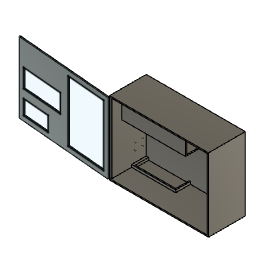
Dispenser (Autodesk Fusion 360 design; units mm, degrees)
Autodesk Fusion 360 part; units mm, degrees
note: some values were not read from the file. Chosen so that the rebuilt part matches the saved one: which bodies a step acts on. Set by a fixed rule: which sketch regions a step uses.
sketch "Sketch1" plane through (0, 0, 0) normal (0, 0, 1) x (1, 0, 0) in component "Box"
  line L0 (0, 0) -> (-404, 0)
  line L1 (-404, 0) -> (-404, 150)
  line L2 (-404, 150) -> (0, 150)
  line L3 (0, 150) -> (0, 0)
  dimension "d1" = 404
  dimension "d2" = 150
  constraint horizontal L0
  constraint vertical L1
  constraint horizontal L2
  constraint vertical L3
  constraint coincident L0.start L3.end
  measures "d1" distance of L0.start L0.end
  measures "d2" distance of L0.start L2.end
extrude "Extrude1" add sketch "Sketch1" along normal blind 298 makes body 1 in component "Box"
shell "Shell1" thickness 5 removed faces 0 bodies 1 in component "Box"
ref_plane "WorkPlane1" through (-202, 5, 149) normal (0, -1, 0) x (1, 0, 0) in component "Box"
split "Split1" by plane through (-202, 5, 149) normal (0, -1, 0) bodies 1 makes body 2 at (-134.6667, 0, 99.3333) in component "Box"
ref_plane "WorkPlane2" through (-202, 75, 293) normal (0, 0, 1) x (1, 0, 0) in component "Box"
ref_plane "WorkPlane3" through (-202, 75, 5) normal (0, 0, -1) x (-1, 0, 0) in component "Box"
ref_plane "WorkPlane4" through (-5, 75, 149) normal (1, 0, 0) x (0, 1, 0) in component "Box"
split "Split2" by plane through (-202, 75, 293) normal (0, 0, 1) and through (-202, 75, 5) normal (0, 0, -1) bodies 2 makes body 3 at (-136.3333, 5, 296.3333) makes body 4 at (-134.6667, 0, 1.6667) in component "Box"
split "Split3" by plane through (-5, 75, 149) normal (1, 0, 0) bodies 2 makes body 5 at (-1.6667, 5, 197) in component "Box"
combine "Combine1" operation add target body 1 tool bodies 3 5 4 in component "Box"
move_body "Move1" bodies 2 to x (-0.996195, 0.087156, 0) y (-0.087156, -0.996195, 0) z (0, 0, 1) at (-806.4627, 35.2109, 0) in component "Box"
sketch "Sketch3" plane through (-3.5046, -40.0579, 0) normal (-0.087156, -0.996195, 0) x (0.996195, -0.087156, 0) in component "Box"
  line L0 (-801.4627, 293) -> (-801.4627, 5)
  line L1 (-801.4627, 5) -> (-402.4627, 5)
  line L2 (-402.4627, 5) -> (-402.4627, 293)
  line L3 (-402.4627, 293) -> (-801.4627, 293)
  line L4 (-581.4627, 273) -> (-422.4627, 273)
  line L5 (-422.4627, 273) -> (-422.4627, 25)
  line L6 (-422.4627, 25) -> (-581.4627, 25)
  line L7 (-581.4627, 25) -> (-581.4627, 273)
  line L8 (-781.4627, 120) -> (-616.4627, 120)
  line L9 (-616.4627, 120) -> (-616.4627, 195)
  line L10 (-616.4627, 195) -> (-781.4627, 195)
  line L11 (-781.4627, 195) -> (-781.4627, 120)
  line L12 (-781.4627, 85) -> (-671.4627, 85)
  line L13 (-671.4627, 85) -> (-671.4627, 25)
  line L14 (-671.4627, 25) -> (-781.4627, 25)
  line L15 (-781.4627, 25) -> (-781.4627, 85)
  dimension "d23" = 159
  dimension "d24" = 248
  dimension "d25" = 165
  dimension "d26" = 75
  dimension "d28" = 20
  dimension "d31" = 20
  dimension "d32" = 20
  dimension "d33" = 110
  dimension "d34" = 60
  dimension "d35" = 20
  dimension "d37" = 20
  dimension "d38" = 35
  constraint horizontal L4
  constraint vertical L5
  constraint horizontal L6
  constraint vertical L7
  constraint horizontal L8
  constraint vertical L9
  constraint horizontal L10
  constraint vertical L11
  constraint horizontal L12
  constraint vertical L13
  constraint horizontal L14
  constraint vertical L15
  measures "d23" distance of L4.start L4.end
  measures "d24" distance of L4.start L6.end
  measures "d25" distance of L8.start L8.end
  measures "d26" distance of L8.start L10.end
  measures "d28" distance of L3 L4
  measures "d31" distance of L0 L11
  measures "d32" distance of L2 L5
  measures "d33" distance of L12.start L12.end
  measures "d34" distance of L12.start L14.end
  measures "d35" distance of L0 L15
  measures "d37" distance of L1 L14
  measures "d38" distance of L8 L12
extrude "Extrude2" cut sketch "Sketch3" against normal up to surface (5 mm away) contours L4 L5 L6 L7 bodies 2 in component "Box"
extrude "Extrude3" cut sketch "Sketch3" against normal up to surface (5 mm away) contours L8 L9 L10 L11 | L12 L13 L14 L15 bodies 2 in component "Box"
sketch "Sketch4" plane through (-399, 0, 0) normal (1, 0, 0) x (0, 1, 0) in component "Box"
  line L0 (5, 5) -> (145, 5)
  line L1 (145, 5) -> (145, 293)
  line L2 (145, 293) -> (5, 293)
  line L3 (5, 293) -> (5, 5)
  line L4 (145, 198) -> (45, 198)
  line L5 (45, 198) -> (45, 193)
  line L6 (45, 193) -> (145, 193)
  line L7 (145, 193) -> (145, 198)
  line L8 (150, 298) -> (0, 298)
  dimension "d44" = 5
  dimension "d45" = 100
  dimension "d46" = 100
  constraint horizontal L4
  constraint vertical L5
  constraint horizontal L6
  constraint vertical L7
  measures "d44" distance of L4.start L6.end
  measures "d45" distance of L4 L8
  measures "d46" distance of L1 L4.end
extrude "Extrude4" add sketch "Sketch4" along normal blind 280 separate body contours L1 L4 L5 L6 L7 makes body 6 in component "Box"
combine "Combine2" operation add target body 1 tool bodies 6 in component "Box"
sketch "Sketch5" plane through (0, 0, 5) normal (0, 0, 1) x (-1, 0, 0) in component "Box"
  line L0 (5, -145) -> (399, -145)
  line L1 (399, -145) -> (399, -5)
  line L2 (399, -5) -> (404, -5)
  line L3 (404, -5) -> (404, 0)
  line L4 (404, 0) -> (5, 0)
  line L5 (5, 0) -> (5, -145)
  line L6 (399, -145) -> (389, -145)
  line L7 (399, -85) -> (389, -85)
  line L8 (389, -85) -> (219, -85)
  line L9 (219, -85) -> (219, -145)
  line L10 (224, -145) -> (224, -90)
  line L11 (224, -90) -> (389, -90)
  line L12 (389, -90) -> (389, -145)
  dimension "d52" = 10
  dimension "d53" = 60
  dimension "d54" = 170
  dimension "d55" = 5
  constraint coincident L0.end L1.start
  constraint perpendicular L1 L6
  constraint coincident L1 L7.start
  constraint perpendicular L1 L7
  constraint coincident L0 L9.end
  constraint perpendicular L0 L9
  constraint coincident L0 L10.start
  constraint perpendicular L0 L10
  constraint perpendicular L6 L12
  measures "d52" distance of L0.end L6.end
  measures "d53" distance of L6.end L7.end
  measures "d54" distance of L7.end L8.end
  measures "d55" distance of L9 L10
extrude "Extrude5" add sketch "Sketch5" along normal blind 10 contours L0 L1 L6 L7 L8 L9 L10 L11 L12 bodies 1 in component "Box"
sketch "Sketch6" plane through (-399, 0, 0) normal (1, 0, 0) x (0, 1, 0) in component "Box"
  line L0 (85, 15) -> (145, 15)
  line L1 (145, 15) -> (145, 193)
  line L2 (145, 193) -> (45, 193)
  line L3 (45, 193) -> (45, 198)
  line L4 (45, 198) -> (145, 198)
  line L5 (145, 198) -> (145, 293)
  line L6 (145, 293) -> (5, 293)
  line L7 (5, 293) -> (5, 5)
  line L8 (5, 5) -> (85, 5)
  line L9 (85, 5) -> (85, 15)
  line L10 (105, 30) -> (95, 30)
  line L11 (95, 30) -> (95, 20)
  line L12 (95, 20) -> (105, 20)
  line L13 (105, 20) -> (105, 30)
  line L14 (95, 90) -> (130, 90)
  line L15 (130, 90) -> (130, 58)
  line L16 (130, 58) -> (95, 58)
  line L17 (95, 58) -> (95, 90)
  line L18 (130, 90) -> (128, 90)
  line L19 (128, 90) -> (128, 88)
  line L20 (128, 88) -> (130, 88)
  line L21 (130, 88) -> (130, 90)
  circle A0 centre (128, 88) radius 1
  line L22 (95, 90) -> (97, 90)
  line L23 (97, 90) -> (97, 88)
  line L24 (97, 88) -> (95, 88)
  line L25 (95, 88) -> (95, 90)
  line L26 (95, 58) -> (97, 58)
  line L27 (97, 58) -> (97, 60)
  line L28 (97, 60) -> (95, 60)
  line L29 (95, 60) -> (95, 58)
  line L30 (130, 58) -> (128, 58)
  line L31 (128, 58) -> (128, 60)
  line L32 (128, 60) -> (130, 60)
  line L33 (130, 60) -> (130, 58)
  circle A1 centre (97, 88) radius 1
  circle A2 centre (97, 60) radius 1
  circle A3 centre (128, 60) radius 1
  dimension "d58" = 10
  dimension "d59" = 10
  dimension "d61" = 25
  dimension "d62" = 40
  dimension "d63" = 35
  dimension "d64" = 32
  dimension "d65" = 50
  dimension "d66" = 2
  dimension "d67" = 2
  dimension "d68" = 2
  dimension "d70" = 2
  dimension "d71" = 2
  dimension "d72" = 2
  dimension "d73" = 2
  dimension "d74" = 2
  dimension "d75" = 2
  dimension "d76" = 2
  dimension "d77" = 2
  dimension "d78" = 2
  constraint horizontal L10
  constraint vertical L11
  constraint horizontal L12
  constraint vertical L13
  constraint horizontal L14
  constraint vertical L15
  constraint horizontal L16
  constraint vertical L17
  constraint horizontal L18
  constraint vertical L19
  constraint horizontal L20
  constraint vertical L21
  constraint coincident L19.end L20.start
  constraint horizontal L22
  constraint vertical L23
  constraint horizontal L24
  constraint vertical L25
  constraint horizontal L26
  constraint vertical L27
  constraint horizontal L28
  constraint vertical L29
  constraint horizontal L30
  constraint vertical L31
  constraint horizontal L32
  constraint vertical L33
  constraint coincident L23.end L24.start
  constraint coincident L27.end L28.start
  constraint coincident L31.end L32.start
  measures "d58" distance of L10.start L10.end
  measures "d59" distance of L10.start L12.end
  measures "d61" distance of L8 L10
  measures "d62" distance of L1 L13
  measures "d63" distance of L14.start L14.end
  measures "d64" distance of L14.start L16.end
  measures "d65" distance of L1 L17
  measures "d66" distance of L14.end L18.end
  measures "d67" distance of L14.end L20.end
  measures "d68" diameter of A0
  measures "d70" distance of L14.start L22.end
  measures "d71" distance of L14.start L24.end
  measures "d72" distance of L16.end L26.end
  measures "d73" distance of L16.end L28.end
  measures "d74" distance of L15.end L30.end
  measures "d75" distance of L15.end L32.end
  measures "d76" diameter of A1
  measures "d77" diameter of A2
  measures "d78" diameter of A3
extrude "Extrude6" add sketch "Sketch6" along normal blind 5 contours L23 L24 A1 | L23 L24 A1 | L19 L20 A0 | L19 L20 A0 | L27 L28 A2 | L27 L28 A2 | L31 L32 A3 | L31 L32 A3 bodies 1 in component "Box"
sketch "Sketch7" plane through (0, 0, 193) normal (0, 0, -1) x (1, 0, 0) in component "Box"
  line L0 (-399, -45) -> (-399, -145)
  line L1 (-399, -145) -> (-119, -145)
  line L2 (-119, -145) -> (-119, -45)
  line L3 (-119, -45) -> (-399, -45)
  line L4 (-389, -90) -> (-382, -90)
  line L5 (-382, -90) -> (-382, -100)
  line L6 (-382, -100) -> (-389, -100)
  line L7 (-389, -100) -> (-389, -90)
  dimension "d81" = 7
  dimension "d82" = 10
  dimension "d83" = 45
  dimension "d84" = 10
  constraint horizontal L4
  constraint vertical L5
  constraint horizontal L6
  constraint vertical L7
  measures "d81" distance of L4.start L4.end
  measures "d82" distance of L4.start L6.end
  measures "d83" distance of L3 L4
  measures "d84" distance of L0 L7
sketch "Sketch8" plane through (0, 0, 198) normal (0, 0, 1) x (-1, 0, 0) in component "Box"
  line L0 (399, -145) -> (399, -45)
  line L1 (399, -45) -> (119, -45)
  line L2 (119, -45) -> (119, -145)
  line L3 (119, -145) -> (399, -145)
  line L4 (399, -145) -> (381, -145)
  line L5 (381, -145) -> (381, -45)
  line L6 (381, -45) -> (399, -45)
  line L7 (399, -45) -> (399, -145)
  dimension "d86" = 18
  dimension "d87" = 100
  constraint horizontal L4
  constraint vertical L5
  constraint horizontal L6
  constraint vertical L7
  constraint coincident L0.start L3.end
  measures "d86" distance of L0.start L4.end
  measures "d87" distance of L0.start L0.end
extrude "Extrude7" cut sketch "Sketch7" against normal up to surface (5 mm away) contours L4 L5 L6 L7 bodies 1 in component "Box"
extrude "Extrude8" add sketch "Sketch8" along normal blind 35 contours L0 L1 L3 L4 L5 L6 L7 bodies 1 in component "Box"
sketch "Sketch9" plane through (-381, 0, 0) normal (1, 0, 0) x (0, 1, 0) in component "Box"
  line L0 (45, 198) -> (145, 198)
  line L1 (145, 198) -> (145, 233)
  line L2 (145, 233) -> (45, 233)
  line L3 (45, 233) -> (45, 198)
  circle A0 centre (95, 215) radius 14
  line L4 (87.7, 198) -> (102.3, 198)
  line L5 (102.3, 198) -> (102.3, 203)
  line L6 (102.3, 203) -> (87.7, 203)
  line L7 (87.7, 203) -> (87.7, 198)
  dimension "d92" = 28
  dimension "d93" = 50
  dimension "d94" = 17
  dimension "d95" = 14.6
  dimension "d96" = 5
  dimension "d97" = 42.7
  constraint horizontal L4
  constraint vertical L5
  constraint horizontal L6
  constraint vertical L7
  constraint coincident L0 L4.start
  measures "d92" diameter of A0
  measures "d93" distance of L1 A0.centre
  measures "d94" distance of L0 A0.centre
  measures "d95" distance of L4.start L4.end
  measures "d96" distance of L4.start L6.end
  measures "d97" distance of L1 L5
extrude "Extrude9" cut sketch "Sketch9" against normal up to surface (18 mm away) contours L0 A0 L4 L5 L6 L7 | A0 L6 | A0 L6 bodies 1 in component "Box"
sketch "Sketch10" plane through (0, 0, 198) normal (0, 0, 1) x (-1, 0, 0) in component "Box"
  line L0 (389, -90) -> (389, -100)
  line L1 (389, -100) -> (382, -100)
  line L2 (382, -100) -> (382, -90)
  line L3 (382, -90) -> (389, -90)
  line L4 (381, -145) -> (381, -102.3)
  line L5 (381, -102.3) -> (399, -102.3)
  line L6 (399, -102.3) -> (399, -87.7)
  line L7 (399, -87.7) -> (381, -87.7)
  line L8 (381, -87.7) -> (381, -45)
  line L9 (381, -45) -> (119, -45)
  line L10 (119, -45) -> (119, -145)
  line L11 (119, -145) -> (381, -145)
  line L12 (381, -45) -> (119, -45)
  line L13 (119, -45) -> (119, -50)
  line L14 (119, -50) -> (381, -50)
  line L15 (381, -50) -> (381, -45)
  dimension "d100" = 5
  constraint horizontal L12
  constraint vertical L13
  constraint horizontal L14
  constraint vertical L15
  constraint coincident L8.end L9.start
  measures "d100" distance of L8.end L14.end
extrude "Extrude10" add sketch "Sketch10" along normal up to surface (35 mm away) contours L8 L9 L10 L12 L13 L14 L15 bodies 1 in component "Box"
move_face "OffsetFaces1" offset -20 1 faces at (-119, 80, 194.6667) on bodies 1 in component "Box"
move_face "OffsetFaces2" offset 15 1 faces at (-393, 80, 233) on bodies 1 in component "Box"
extrude "Extrude11" add 1 faces at (-399, 92.9024, 212.4305) along direction (1, 0, 0) blind 18 on bodies 1 bodies 1 in component "Box"
sketch "Sketch11" plane through (-381, 0, 0) normal (1, 0, 0) x (0, 1, 0) in component "Box"
  line L0 (50, 198) -> (145, 198)
  line L1 (145, 198) -> (145, 248)
  line L2 (145, 248) -> (50, 248)
  line L3 (50, 248) -> (50, 198)
  circle A0 centre (95, 230) radius 14
  line L4 (87.7, 218) -> (102.3, 218)
  line L5 (102.3, 218) -> (102.3, 213)
  line L6 (102.3, 213) -> (87.7, 213)
  line L7 (87.7, 213) -> (87.7, 218)
  dimension "d107" = 28
  dimension "d108" = 50
  dimension "d109" = 32
  dimension "d110" = 14.6
  dimension "d111" = 5
  dimension "d112" = 42.7
  dimension "d113" = 15
  constraint horizontal L4
  constraint vertical L5
  constraint horizontal L6
  constraint vertical L7
  measures "d107" diameter of A0
  measures "d108" distance of L1 A0.centre
  measures "d109" distance of L0 A0.centre
  measures "d110" distance of L4.start L4.end
  measures "d111" distance of L4.start L6.end
  measures "d112" distance of L1 L5
  measures "d113" distance of L0 L6
extrude "Extrude12" cut sketch "Sketch11" against normal up to surface (18 mm away) contours A0 L4 | A0 L4 | A0 L4 L5 L6 L7 bodies 1 in component "Box"
extrude "Extrude13" cut 1 faces at (-384.3333, 93.3333, 198) along direction (0, 0, 1) up to surface (15 mm away) on bodies 1 bodies 1 in component "Box"
component "Box" placed x (1, 0, 0) y (0, 1, 0) z (0, 0, 1) at (4.5931, -0.4018, -1.729)
equation "d1 = BoxLength"
equation "d2 = BoxWidth"
equation "BoxHeight = 298 mm"
equation "WallThickness = 5 mm"
equation "BoxWidth = 150 mm"
equation "BoxLength = 404 mm"
equation "d7 = BoxHeight"
equation "d9 = WallThickness"
equation "d10 = -WallThickness"
equation "d11 = -WallThickness"
equation "d12 = -WallThickness"
equation "d13 = -WallThickness"
equation "HingeRadius = HingeThickness * 2"
equation "Gap = HingeThickness * 0.5 / 1.3"
equation "HingeThickness = 3 mm"
equation "d28 = ( BoxHeight - ( 2 * WallThickness ) - 248 mm ) / 2"
equation "d37 = ( BoxHeight - ( 2 * WallThickness ) - 248 mm ) / 2"
equation "d44 = WallThickness"
